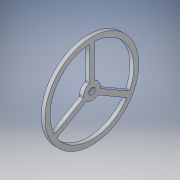
# Autodesk Inventor part: Rueda_triciclo
Saved by Autodesk Inventor 2019 (Build 230136000, 136)
## iProperties
Created: 2019-11-14
Part Number: Rueda_triciclo
Material: Aluminum 6061
Document SubType Name: Modeling
Designer: Domenico
Density: 2.7 g/cm^3
Appearance: Aluminum - Flat
Mass: 289.941 g
Surface Area: 410.48 cm^2
Volume: 107.386 cm^3
D_eje: 15.000 mm
Author: Domenico
Autodesk Inventor part; units mm, degrees
ref_plane "YZ Plane" through (0, 0, 0) normal (1, 0, 0) x (0, 1, 0)
ref_plane "XZ Plane" through (0, 0, 0) normal (0, 1, 0) x (-1, 0, 0)
ref_plane "XY Plane" through (0, 0, 0) normal (0, 0, 1) x (1, 0, 0)
sketch "Sketch1" plane through (0, 0, 0) normal (1, 0, 0) x (0, 1, 0)
  circle A0 centre (0, 0) radius 7.5
  circle A1 centre (0, 0) radius 111.9
  dimension "D_eje" = 15
  dimension "d1" = 223.8
  constraints: 2 centre point, 2 coincident
  measures "D_eje" diameter of A0
  measures "d1" diameter of A1
extrude "Extrusion1" add sketch "Sketch1" along normal blind 9
sketch "Sketch2" plane through (9, 0, 0) normal (1, 0, 0) x (0, 0, -1)
  line L0 (6, 19.0264) -> (6, 99.7197)
  line L1 (0, -188.1875) -> (0, 173.8632) construction
  arc A0 (0, 19.95) -> (-13.4773, 14.7093) centre (0, 0) ccw construction
  circle A1 centre (0, 0) radius 7.5 construction
  arc A2 (0, 99.9) -> (86.5159, -49.95) centre (0, 0) ccw construction
  line L2 (181.1282, 0) -> (-189.3983, 0) construction
  arc A3 (6, 19.0264) -> (0, 19.95) centre (0, 0) ccw construction
  arc A4 (-19.95, 0) -> (0, -19.95) centre (0, 0) ccw construction
  arc A5 (0, -19.95) -> (17.2772, -9.975) centre (0, 0) ccw construction
  arc A6 (19.95, 0) -> (6, 19.0264) centre (0, 0) ccw
  line L3 (0, 0) -> (86.5159, -49.95) construction
  line L4 (19.4773, -4.317) -> (89.3598, -44.6637)
  arc A7 (-13.4773, 14.7093) -> (-19.95, 0) centre (0, 0) ccw construction
  arc A8 (19.4773, -4.317) -> (19.95, 0) centre (0, 0) ccw
  arc A9 (17.2772, -9.975) -> (19.4773, -4.317) centre (0, 0) ccw construction
  arc A10 (6, 99.7197) -> (0, 99.9) centre (0, 0) ccw construction
  arc A11 (86.5159, -49.95) -> (89.3598, -44.6637) centre (0, 0) ccw construction
  arc A12 (89.3598, -44.6637) -> (6, 99.7197) centre (0, 0) ccw
  line L5 (-19.4773, -4.317) -> (-89.3598, -44.6637)
  arc A13 (-6, 99.7197) -> (-89.3598, -44.6637) centre (0, 0) ccw
  line L6 (-6, 19.0264) -> (-6, 99.7197)
  arc A14 (-9.975, 17.2772) -> (-19.4773, -4.317) centre (0, 0) ccw
  line L7 (13.4773, -14.7093) -> (83.3598, -55.056)
  arc A15 (-83.3598, -55.056) -> (83.3598, -55.056) centre (0, 0) ccw
  line L8 (-13.4773, -14.7093) -> (-83.3598, -55.056)
  arc A16 (-9.975, -17.2772) -> (13.4773, -14.7093) centre (0, 0) ccw
  point P0 (-6, -19.0264)
  point P1 (19.4773, 4.317)
  dimension "d4" = 6
  dimension "d7" = 39.9
  dimension "d8" = 199.8
  dimension "d10" = 120
  dimension "d11" = 6
  dimension "d14" = 360
  constraints: 33 point on circle, 16 centre point, 14 end point, 9 point on line, 3 coincident, 1 vertical, 37 other
  measures "d4" distance between parallel lines of L1 L0
  measures "d7" diameter of A0
  measures "d8" diameter of A2
  measures "d10" angle of L3 L0
  measures "d11" distance between parallel lines of L3 L4
extrude "Extrusion2" cut sketch "Sketch2" against normal blind 9
pattern_circular "Circular Pattern1" count 3 over 360 about axis through (-10, 0, 0) along (1, 0, 0) of "Extrusion2"
fillet "Fillet1" radius 2 12 edges at (4.5, -14.7093, -13.4773) (4.5, -14.7093, 13.4773) (4.5, -55.056, 83.3598) (4.5, -55.056, -83.3598) (4.5, -44.6637, -89.3598) (4.5, 99.7197, -6) (4.5, -4.317, -19.4773) (4.5, 19.0264, -6) (4.5, 19.0264, 6) (4.5, -4.317, 19.4773) (4.5, 99.7197, 6) (4.5, -44.6637, 89.3598)
body "Solid1"
